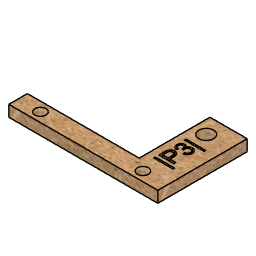
P3 (Autodesk Fusion 360 design; units mm, degrees)
Autodesk Fusion 360 part; units mm, degrees
sketch "Esboço1" plane through (0, 0, 0) normal (0, 1, 0) x (1, 0, 0)
  line L0 (0, 0) -> (40, 0)
  line L1 (0, 5) -> (0, 0)
  circle A0 centre (6, 2.5) radius 1.5
  circle A1 centre (33.5, 2.5) radius 1.5
  line L2 (0, 5) -> (30, 5)
  line L3 (30, 5) -> (30, 24)
  line L4 (30, 24) -> (40, 24)
  line L5 (40, 24) -> (40, 0)
  circle A2 centre (33.5, 19.5) radius 2
  dimension "d3" = 3
  dimension "d4" = 2.5
  dimension "d5" = 6
  dimension "d6" = 3
  dimension "d7" = 2.5
  dimension "d19" = 5
  dimension "d20" = 40
  dimension "d21" = 27.5
  dimension "d22" = 10
  dimension "d23" = 4
  dimension "d24" = 17
  dimension "d25" = 24
  dimension "d26" = 6.5
  constraint horizontal L0
  constraint vertical L1
  constraint coincident L0.start L1.end
  constraint perpendicular L1 L2
  constraint perpendicular L2 L3
  constraint perpendicular L3 L4
  measures "d3" diameter of A0
  measures "d4" distance of L0 A0.centre
  measures "d5" distance of L1 A0.centre
  measures "d6" diameter of A1
  measures "d7" distance of L0 A1.centre
  measures "d19" distance of L0 L2
  measures "d20" distance of L1 L5
  measures "d21" distance of A0.centre A1.centre
  measures "d22" distance of L3 L5
  measures "d23" diameter of A2
  measures "d24" vertical distance of A1.centre A2.centre
  measures "d25" distance of L0 L4
  measures "d26" distance of L5 A2.centre
extrude "Extrusão1" add sketch "Esboço1" along normal blind 3
sketch "Esboço2" plane through (0, 3, 0) normal (0, 1, 0) x (-1, 0, 0)
  circle A0 centre (-33.5, -2.5) radius 1.5
  circle A1 centre (-6, -2.5) radius 1.5
  line L0 (0, -5) -> (0, 0)
  line L1 (0, 0) -> (-40, 0)
  line L2 (-38.9251, -7.3351) -> (-38.9251, -15.3856) construction
  line L3 (-38.9251, -15.3856) -> (-28.9724, -15.3856) construction
  line L4 (-28.9724, -15.3856) -> (-28.9724, -7.3351) construction
  line L5 (-28.9724, -7.3351) -> (-38.9251, -7.3351) construction
  line L6 (-40, 0) -> (-40, -24)
  line L7 (-40, -24) -> (-30, -24)
  line L8 (-30, -24) -> (-30, -5)
  line L9 (-30, -5) -> (0, -5)
  circle A2 centre (-33.5, -19.5) radius 2
  dimension "d15" = 4
  text T0 "|P3|" font "Arial" height 4 align centre middle in box 8.0505 x 9.9527 at (-38.9251, -7.3351) x (0, -1) y (1, 0) spacing 1
extrude "Extrusão2" cut sketch "Esboço2" against normal blind 1 text T0
